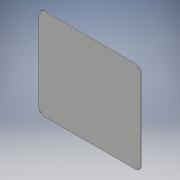
# Autodesk Inventor part: right_panel_atx
Saved by Autodesk Inventor 2018 (Build 220112000, 112)
## iProperties
Created: 2021-04-25
Part Number: right_panel_atx
Material: Generic
Document SubType Name: Modeling
Designer: gisen
Density: 1 g/cm^3
Appearance: Default
Author: gisen
Autodesk Inventor part; units mm, degrees
ref_plane "YZ Plane" through (0, 0, 0) normal (1, 0, 0) x (0, 1, 0)
ref_plane "XZ Plane" through (0, 0, 0) normal (0, 1, 0) x (-1, 0, 0)
ref_plane "XY Plane" through (0, 0, 0) normal (0, 0, 1) x (1, 0, 0)
sketch "Sketch1" plane through (0, 0, 0) normal (0, 1, 0) x (-1, 0, 0)
  line L0 (-192.5, -190) -> (192.5, -190)
  line L1 (212.5, -170) -> (212.5, 170)
  line L2 (192.5, 190) -> (-192.5, 190)
  line L3 (-212.5, 170) -> (-212.5, -170)
  line L4 (-212.5, -190) -> (212.5, 190) construction
  line L5 (212.5, -190) -> (-212.5, 190) construction
  circle A0 centre (202.5, 180) radius 2.25
  circle A1 centre (202.5, -180) radius 2.25
  circle A2 centre (-202.5, 180) radius 2.25
  circle A3 centre (-202.5, -180) radius 2.25
  arc A4 (-192.5, 190) -> (-212.5, 170) centre (-192.5, 170) ccw
  arc A5 (192.5, -190) -> (212.5, -170) centre (192.5, -170) ccw
  arc A6 (212.5, 170) -> (192.5, 190) centre (192.5, 170) ccw
  arc A7 (-212.5, -170) -> (-192.5, -190) centre (-192.5, -170) ccw
  point P0 (0, 0)
  dimension "d0" = 380
  dimension "d1" = 425
  dimension "d4" = 4.5
  dimension "d5" = 4.5
  dimension "d6" = 10
  dimension "d7" = 10
  dimension "d8" = 10
  dimension "d9" = 10
  dimension "d10" = 4.5
  dimension "d11" = 4.5
  dimension "d12" = 10
  dimension "d13" = 10
  dimension "d14" = 10
  dimension "d15" = 10
  dimension "d16" = 20
  dimension "d17" = 20
  dimension "d18" = 20
  dimension "d19" = 20
  constraints: 12 end point, 8 centre point, 8 point on circle, 8 point on line, 8 tangent, 2 midpoint, 2 parallel, 1 horizontal, 1 perpendicular
  measures "d0" distance of L5.end L4.start
  measures "d1" distance of L4.end L5.end
  measures "d4" diameter of A0
  measures "d5" diameter of A1
  measures "d6" distance from line of L1 A0.centre
  measures "d7" distance from line of A0.centre L2
  measures "d8" distance from line of A1.centre L1
  measures "d9" distance from line of L0 A1.centre
  measures "d10" diameter of A2
  measures "d11" diameter of A3
  measures "d12" distance from line of L2 A2.centre
  measures "d13" distance from line of L3 A2.centre
  measures "d14" distance from line of L3 A3.centre
  measures "d15" distance from line of L0 A3.centre
  measures "d16" radius of A4
  measures "d17" radius of A5
  measures "d18" radius of A6
  measures "d19" radius of A7
extrude "Extrusion2" add sketch "Sketch1" along normal blind 3
equation "\"d8\" = d6"
equation "\"d9\" = d7"
equation "\"d10\" = d4"
equation "\"d11\" = d5"
equation "\"d12\" = d7"
equation "\"d13\" = d6"
equation "\"d14\" = d13"
equation "\"d15\" = d8"
body "Solid2"
